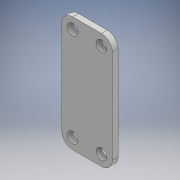
# Autodesk Inventor part: mocowanie do podstawy2
Saved by Autodesk Inventor 2017.3 (Build 213256000, 256)
## iProperties
Created: 2019-03-17
Part Number: mocowanie do podstawy2
Material: Ogólny
Document SubType Name: Modeling
Designer: legox
Density: 1 g/cm^3
Appearance: Domyślna
Author: legox
Autodesk Inventor part; units mm, degrees
ref_plane "YZ Plane" through (0, 0, 0) normal (1, 0, 0) x (0, 1, 0)
ref_plane "XZ Plane" through (0, 0, 0) normal (0, 1, 0) x (-1, 0, 0)
ref_plane "XY Plane" through (0, 0, 0) normal (0, 0, 1) x (1, 0, 0)
sketch "Szkic1" plane through (0, 0, 0) normal (0, 1, 0) x (-1, 0, 0)
  circle A0 centre (4, 13) radius 1.5
  circle A1 centre (-4, 13) radius 1.5
  circle A2 centre (4, -13) radius 1.5
  circle A3 centre (-4, -13) radius 1.5
  line L0 (4, 16) -> (-4, 16)
  line L1 (-7, 13) -> (-7, -13)
  line L2 (-4, -16) -> (4, -16)
  line L3 (7, -13) -> (7, 13)
  arc A4 (7, 13) -> (4, 16) centre (4, 13) ccw
  arc A5 (4, -16) -> (7, -13) centre (4, -13) ccw
  arc A6 (-7, -13) -> (-4, -16) centre (-4, -13) ccw
  arc A7 (-4, 16) -> (-7, 13) centre (-4, 13) ccw
  point P0 (0, 0)
  point P1 (-7, -16)
  point P2 (-7, 16)
  point P3 (7, -16)
  dimension "d0" = 3
  dimension "d1" = 13
  dimension "d2" = 4
  dimension "d4" = 14
  dimension "d5" = 32
  dimension "d6" = 3
  constraints: 8 centre point, 8 end point, 8 point on circle, 8 tangent, 6 point on line, 3 equal radius, 2 parallel, 1 horizontal, 1 perpendicular
  measures "d0" diameter of A0
  measures "d1" vertical distance of point (0, 0) A0.centre
  measures "d2" horizontal distance of A0.centre point (0, 0)
  measures "d4" distance of point (7, -16) point (-7, -16)
  measures "d5" distance of point (-7, -16) point (-7, 16)
  measures "d6" radius of A4
extrude "Wyciągnięcie proste1" add sketch "Szkic1" along normal blind 1.6
